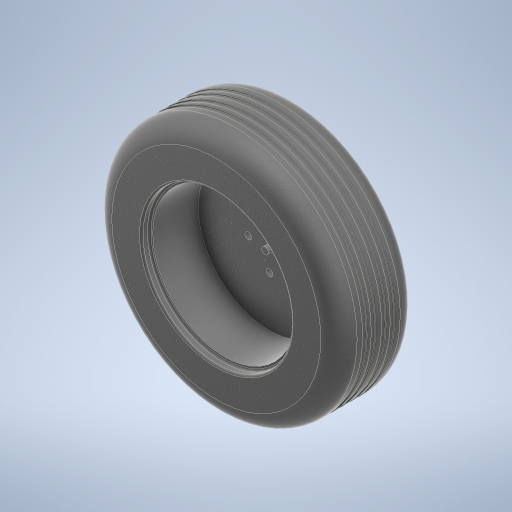
# Autodesk Inventor part: wheel
Saved by Autodesk Inventor 2023 (Build 270158000, 158)
## iProperties
Created: 2024-02-05
Part Number: wheel
Material: 고무
Document SubType Name: Modeling
Designer: ps737
Density: 0.93 g/cm^3
Appearance: 암회색
Author: ps737
Autodesk Inventor part; units mm, degrees
ref_plane "YZ Plane" through (0, 0, 0) normal (1, 0, 0) x (0, 1, 0)
ref_plane "XZ Plane" through (0, 0, 0) normal (0, 1, 0) x (-1, 0, 0)
ref_plane "XY Plane" through (0, 0, 0) normal (0, 0, 1) x (1, 0, 0)
sketch "스케치1" plane through (0, 0, 0) normal (0, 0, 1) x (1, 0, 0)
  circle A0 centre (0, 0) radius 270
  circle A1 centre (0, 0) radius 165
  dimension "d0" = 540
  dimension "d1" = 330
  constraints: 2 centre point, 2 coincident
  measures "d0" diameter of A0
  measures "d1" diameter of A1
extrude "돌출1" add sketch "스케치1" along normal mid plane 175
extrude "돌출2" add sketch "스케치1" along normal mid plane 140 contours A1
fillet "모깎기1" radius 4 2 edges at (-165, 0, 87.5) (-165, 0, 70)
fillet "모깎기2" radius 40 2 edges at (-270, 0, 87.5) (-270, 0, -87.5)
sketch "스케치2" plane through (0, 0, 0) normal (0, 0, 1) x (1, 0, 0)
  circle A0 centre (0, 0) radius 25
  circle A1 centre (0, 47.0427) radius 7.5
  circle A2 centre (-47.0427, 0) radius 7.5
  circle A3 centre (0, -47.0427) radius 7.5
  circle A4 centre (47.0427, 0) radius 7.5
  dimension "d8" = 50
  dimension "d9" = 15
  dimension "d12" = 360
  constraints: 5 centre point, 1 coincident, 9 other
  measures "d8" diameter of A0
  measures "d9" diameter of A1
extrude "돌출3" add sketch "스케치2" along normal mid plane 150 contours A0
extrude "돌출4" cut sketch "스케치2" along normal mid plane 150 contours A1 | A2 | A3 | A4
sketch "스케치4" plane through (0, 0, 0) normal (1, 0, 0) x (0, 1, 0)
  line L0 (270, -47.5) -> (270, 47.5) projected
  line L1 (270, 35.3814) -> (267.8692, 35.3814)
  line L2 (267.8692, 35.3814) -> (267.8692, 25.3814)
  line L3 (267.8692, 25.3814) -> (270, 25.3814)
  line L4 (270, 16.4038) -> (267.8692, 16.4038)
  line L5 (267.8692, 16.4038) -> (267.8692, 6.4038)
  line L6 (267.8692, 6.4038) -> (270, 6.4038)
  line L7 (280.9878, 0) -> (263.4352, 0)
  line L8 (270, -35.3814) -> (267.8692, -35.3814)
  line L9 (267.8692, -35.3814) -> (267.8692, -25.3814)
  line L10 (267.8692, -25.3814) -> (270, -25.3814)
  line L11 (267.8692, -6.4038) -> (270, -6.4038)
  line L12 (267.8692, -16.4038) -> (267.8692, -6.4038)
  line L13 (270, -16.4038) -> (267.8692, -16.4038)
  line L14 (0, 108.3744) -> (0, -123.7727) construction
  point P0 (0, 0)
  dimension "d20" = 10
  dimension "d21" = 10
  constraints: 28 end point, 8 symmetric about line, 4 perpendicular, 3 horizontal, 1 vertical
  measures "d20" distance of L1.end L2.end
  measures "d21" distance of L5.start L6.start
revolve "회전1" cut sketch "스케치4" angle 360 about axis through (0, 0, 108.3744) along (0, 0, -1)
sketch "스케치5" plane through (0, 0, 70) normal (0, 0, 1) x (1, 0, 0)
  circle A0 centre (0, 0) radius 157.111
  constraints: 1 centre point, 1 coincident
extrude "돌출5" cut sketch "스케치5" along normal blind 50 and the other way blind 100
sketch "스케치8" plane through (0, 0, -30) normal (0, 0, 1) x (1, 0, 0)
  circle A0 centre (0, 0) radius 7.5
  dimension "d31" = 15
  constraints: 1 centre point, 1 coincident
  measures "d31" diameter of A0
extrude "돌출6" add sketch "스케치8" along normal blind 10
